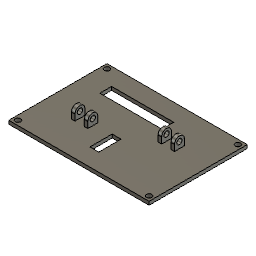
RPi+Board+Cover (Autodesk Fusion 360 design; units mm, degrees)
Autodesk Fusion 360 part; units mm, degrees
note: some values were not read from the file. Set by a fixed rule: which face or edge a step refers to.
sketch "Sketch2" plane through (0, 0, 0) normal (0, 1, 0) x (1, 0, 0)
  line L0 (-60, 42) -> (60, 42)
  line L1 (60, 42) -> (60, -42)
  line L2 (60, -42) -> (-60, -42)
  line L3 (-60, -42) -> (-60, 42)
  line L4 (-41, 27) -> (12, 27)
  line L5 (12, 27) -> (12, 17)
  line L6 (12, 17) -> (-41, 17)
  line L7 (-41, 17) -> (-41, 27)
  line L8 (-5.5, -8) -> (2, -8)
  line L9 (2, -8) -> (2, -27)
  line L10 (2, -27) -> (-5.5, -27)
  line L11 (-5.5, -27) -> (-5.5, -8)
  circle A0 centre (-56, 38) radius 2.25
  circle A1 centre (56, 38) radius 2.25
  circle A2 centre (56, -38) radius 2.25
  circle A3 centre (-56, -38) radius 2.25
  line L12 (-56, 38) -> (-56, -38) construction
  line L13 (-56, -38) -> (56, -38) construction
  line L14 (56, -38) -> (56, 38) construction
  line L15 (56, 38) -> (-56, 38) construction
  dimension "d21" = 120
  dimension "d22" = 60
  dimension "d23" = 84
  dimension "d24" = 42
  dimension "d25" = 19
  dimension "d26" = 15
  dimension "d27" = 10
  dimension "d28" = 53
  dimension "d29" = 15
  dimension "d30" = 7.5
  dimension "d31" = 54.5
  dimension "d32" = 19
  dimension "d40" = 4
  dimension "d41" = 4
  dimension "d42" = 4
  dimension "d43" = 4
  dimension "d44" = 4.5
  constraint horizontal L0
  constraint vertical L1
  constraint horizontal L2
  constraint vertical L3
  constraint horizontal L4
  constraint vertical L5
  constraint horizontal L6
  constraint vertical L7
  constraint horizontal L8
  constraint vertical L9
  constraint horizontal L10
  constraint vertical L11
  constraint equal A0 A1
  constraint equal A0 A2
  constraint equal A0 A3
  constraint coincident A0.centre L12.start
  constraint coincident A3.centre L12.end
  constraint coincident A2.centre L13.end
  constraint horizontal L13
  constraint coincident A1.centre L14.end
  constraint parallel L13 L15
  constraint perpendicular L12 L15
  constraint perpendicular L14 L15
  measures "d21" distance of L0.start L0.end
  measures "d22" distance of origin L1
  measures "d23" distance of L0.start L2.end
  measures "d24" distance of origin L0
  measures "d25" distance of L3 L7
  measures "d26" distance of L0 L4
  measures "d27" distance of L4.start L6.end
  measures "d28" distance of L4.start L4.end
  measures "d29" distance of L2 L10
  measures "d30" distance of L8.start L8.end
  measures "d31" distance of L3 L11
  measures "d32" distance of L8.start L10.end
  measures "d40" distance of L0 L15
  measures "d41" distance of L2 L13
  measures "d42" distance of L3 L12
  measures "d43" distance of L1 L14
  measures "d44" diameter of A0
extrude "Extrude1" add sketch "Sketch2" along normal blind 3
ref_plane "WorkPlane1" through (-20, 0, 0) normal (1, 0, 0) x (0, 1, 0)
sketch "Sketch6" plane through (-20, 0, 0) normal (1, 0, 0) x (0, 0, -1)
  circle A0 centre (9.9499, 8.25) radius 4.25
  line L0 (5.6999, 8.25) -> (9.9499, 8.25) construction
  line L1 (9.9499, 8.25) -> (14.1999, 8.25) construction
  circle A1 centre (9.9499, 8.25) radius 2.25
  line L2 (5.6999, 8.25) -> (5.6999, 3)
  line L3 (14.1999, 8.25) -> (14.1999, 3)
  line L4 (-42, 3) -> (42, 3)
  line L5 (9.9499, 8.25) -> (9.9499, 4) construction
  point P0 (0, 3)
  dimension "d33" = 4.5
  dimension "d34" = 8.5
  dimension "d45" = 10
  dimension "d54" = 1
  constraint coincident A0 L0.start
  constraint coincident A0.centre L0.end
  constraint horizontal L0
  constraint coincident A0 L1.end
  constraint parallel L0 L1
  constraint tangent A0 L2
  constraint perpendicular L1 L3
  constraint coincident L2.end L4
  constraint coincident L3.end L4
  constraint coincident L1.end L3.start
  constraint coincident A0 L5.end
  constraint perpendicular L1 L5
  constraint midpoint L4 P0
  measures "d33" diameter of A1
  measures "d34" diameter of A0
  measures "d45" distance of L5.end P0
  measures "d54" distance of L4 L5.end
extrude "Extrude5" add sketch "Sketch6" against normal blind 14
ref_plane "WorkPlane3" through (-27, 0, 0) normal (1, 0, 0) x (0, 1, 0)
sketch "Sketch7" plane through (-27, 0, 0) normal (1, 0, 0) x (0, 0, -1)
  circle A0 centre (9.9499, 8.25) radius 2.25
  arc A1 (14.1999, 8.25) -> (5.6999, 8.25) centre (9.9499, 8.25) ccw
  line L0 (5.6999, 8.25) -> (5.6999, 3)
  line L1 (5.6999, 3) -> (14.1999, 3)
  line L2 (14.1999, 3) -> (14.1999, 8.25)
extrude "Extrude6" cut sketch "Sketch7" along normal mid plane 8
pattern_linear "R-Pattern1" count 2 spacing 20 along (0, 0, 1) count 2 spacing 54 along (1, 0, 0) of "Extrude5", "Extrude6"
extrude "Extrude7" cut 1 faces at (-34, 4.0021, -10.0059) along direction (1, 0, 0) up to surface (14 mm away)
extrude "Extrude8" cut 1 faces at (20, 4.0021, 9.9941) along direction (1, 0, 0) up to surface (14 mm away)
equation "d3 = -20.00 mm"
equation "d22 = d21 / 2"
equation "d24 = d23 / 2"
equation "d34 = d33 + 4 mm"
equation "d35 = -14.00 mm"
equation "d37 = d3 + ( d35 / 2 mm ) * 1 mm"
equation "d41 = d40"
equation "d42 = d40"
equation "d43 = d42"
equation "d48 = 2 * d45"
equation "d49 = d37 * -2"
